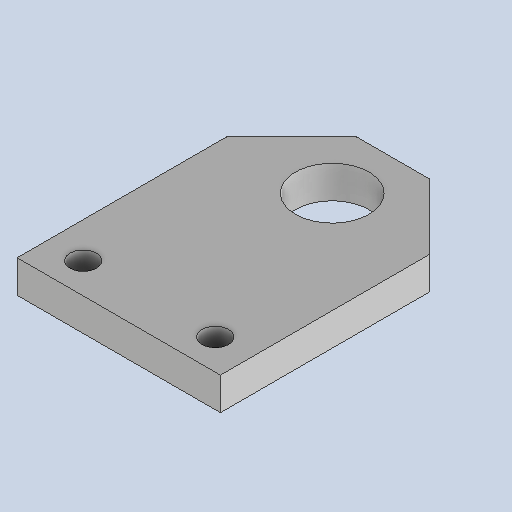
# Autodesk Inventor part: Part1
Saved by Autodesk Inventor 2025 (Build 290162010, 162A)
## iProperties
Created: 2024-06-21
Part Number: Part1
Material: Stainless Steel
Document SubType Name: Sheet Metal
Designer: admin
Density: 8 g/cm^3
Sheet Metal Rule: AISI304 2mm Die16
Appearance: Default
Author: admin
Autodesk Inventor part; units mm, degrees
ref_plane "YZ Plane" through (0, 0, 0) normal (1, 0, 0) x (0, 1, 0)
ref_plane "XZ Plane" through (0, 0, 0) normal (0, 1, 0) x (-1, 0, 0)
ref_plane "XY Plane" through (0, 0, 0) normal (0, 0, 1) x (1, 0, 0)
sketch "Sketch1" plane through (0, 0, 0) normal (0, 0, 1) x (1, 0, 0)
  line L0 (-50, 135) -> (50, 135)
  line L1 (50, 135) -> (50, 0)
  line L2 (50, 0) -> (-50, 0)
  line L3 (-50, 0) -> (-50, 135)
  circle A0 centre (0, 105) radius 18.05
  line L4 (-18, 135) -> (-50, 103)
  line L5 (18, 135) -> (50, 103)
  circle A1 centre (-32.5, 15) radius 6.5
  circle A2 centre (32.5, 15) radius 6.5
  line L6 (-32.5, 15) -> (32.5, 15) construction
  point P0 (0, 0)
  point P1 (0, 0)
  point P2 (0, 15)
  dimension "d0" = 100
  dimension "d1" = 36.1
  dimension "d2" = 105
  dimension "d3" = 32
  dimension "d4" = 135
  dimension "d6" = 45
  dimension "d7" = 13
  dimension "d8" = 65
  dimension "d9" = 15
  measures "d0" distance of L1.end L2.end
  measures "d1" diameter of A0
  measures "d2" distance of point (0, 0) A0.centre
  measures "d3" distance of L0.start L4.end
  measures "d4" distance of L2.end L0.start
  measures "d6" angle of L3 L4
  measures "d7" diameter of A1
  measures "d8" distance of L6.end L6.start
  measures "d9" distance between parallel lines of L2 L6
extrude "Plate1" add sketch "Sketch1" along normal blind 16 contours L0 L5 L1 L2 L3 L4
equation "\"d10\" = Thickness"
equation "\"BendReliefWidth\" = Thickness"
equation "\"BendReliefDepth\" = 0.5 * Thickness"
equation "\"CornerReliefSize\" = 4 * Thickness"
equation "\"MinimumRemnant\" = 2 * Thickness"
equation "\"TransitionRadius\" = BendRadius"
equation "\"JacobiRadiusSize\" = BendRadius"
equation "\"GapSize\" = Thickness"
equation "\"Thickness\" = 16"
equation "\"BendRadius\" = 2.75"
body "Solid1"
